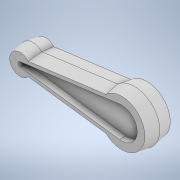
# Autodesk Inventor part: Ch3 Part 2
Saved by Autodesk Inventor 2020 (Build 240168000, 168)
## iProperties
Created: 2021-02-04
Part Number: Ch3 Part 2
Material: Generic
Document SubType Name: Modeling
Designer: austi
Density: 1 g/cm^3
Appearance: Default
Author: austi
Autodesk Inventor part; units mm, degrees
ref_plane "YZ Plane" through (0, 0, 0) normal (1, 0, 0) x (0, 1, 0)
ref_plane "XZ Plane" through (0, 0, 0) normal (0, 1, 0) x (-1, 0, 0)
ref_plane "XY Plane" through (0, 0, 0) normal (0, 0, 1) x (1, 0, 0)
sketch "Sketch1" plane through (0, 0, 0) normal (0, 0, 1) x (1, 0, 0)
  line L0 (-40.64, 0) -> (154.94, 0)
  line L1 (0, -35.56) -> (0, 35.56)
  arc A0 (8.901936, 9.057899) -> (8.901936, -9.057899) centre (0, 0) ccw
  arc A1 (84.799479, -19.05) -> (84.799479, 19.05) centre (101.6, 0) ccw
  line L2 (8.901936, 9.057899) -> (84.799479, 19.05)
  line L3 (8.901936, -9.057899) -> (84.799479, -19.05)
  dimension "d1" = 25.4
  dimension "d3" = 50.8
  dimension "d4" = 15
  dimension "d5" = 38.1
  dimension "d6" = 101.6
  constraints: 4 end point, 4 point on circle, 2 centre point, 2 vertical alignment, 1 coincident, 1 horizontal alignment
  measures "d1" diameter of A0
  measures "d3" diameter of A1
  measures "d4" angle of L3 L2
  measures "d5" distance of L3.end L2.end
  measures "d6" distance of A1.centre point (0, 0)
sketch "Sketch1 outline for Extrusion1" plane through (0, 0, 0) normal (0, 0, 1) x (1, 0, 0)
  arc A0 (8.901936, 9.057899) -> (8.901936, -9.057899) centre (0, 0) ccw
  line L0 (84.799479, 19.05) -> (8.901936, 9.057899)
  arc A1 (84.799479, -19.05) -> (84.799479, 19.05) centre (101.6, 0) ccw
  line L1 (8.901936, -9.057899) -> (84.799479, -19.05)
extrude "Extrusion1" add sketch "Sketch1 outline for Extrusion1" along normal mid plane 25.4 draft -10
sketch "Sketch2" plane through (0, 0, 12.7) normal (0, 0, 1) x (1, 0, 0)
  line L0 (0, 2.296768) -> (99.571808, 15.405645)
  line L1 (8.044726, 6.686369) -> (85.785782, 16.921173)
  line L2 (0, -35.56) -> (0, 35.56)
  line L3 (-40.64, 0) -> (154.94, 0)
  line L4 (0, -2.296768) -> (99.571808, -15.405645)
  arc A0 (0, 2.296768) -> (0, -2.296768) centre (0.302375, 0) ccw
  arc A1 (99.571808, -15.405645) -> (99.571808, 15.405645) centre (101.6, 0) ccw
  arc A2 (85.785782, -16.921173) -> (85.785782, 16.921173) centre (101.6, 0) ccw
  point P0 (0, 0)
  point P1 (8.355059, 3.396732)
  point P2 (8.355059, -3.396732)
  dimension "d10" = 3.302
  constraints: 6 point on line, 4 end point, 4 point on circle, 2 centre point, 2 symmetric about line, 2 tangent, 1 concentric, 1 parallel
  measures "d10" distance between parallel lines of L1 L0
extrude "Extrusion2" cut sketch "Sketch2" against normal blind 6.35
sketch "Sketch3" plane through (0, 0, -12.7) normal (0, 0, -1) x (-1, 0, 0)
  arc A0 (0, -2.296768) -> (0, 2.296768) centre (-0.302375, 0) ccw
  arc A1 (0, -2.296768) -> (0, 2.296768) centre (-0.302375, 0) ccw
  line L0 (-99.571808, -15.405645) -> (0, -2.296768)
  line L1 (0, 2.296768) -> (-99.571808, 15.405645)
  arc A2 (-99.571808, 15.405645) -> (-99.571808, -15.405645) centre (-101.6, 0) ccw
  arc A3 (-99.571808, 15.405645) -> (-99.571808, -15.405645) centre (-101.6, 0) ccw
  line L2 (0, -2.296768) -> (-99.571808, -15.405645)
  line L3 (-85.785782, 16.921173) -> (-8.044726, 6.686369)
  point P0 (0, 0)
  point P1 (0, 2.296768)
  constraints: 6 end point, 5 point on circle, 2 centre point, 2 coincident, 1 collinear, 1 parallel, 1 point on line
extrude "Extrusion3" cut sketch "Sketch3" against normal blind 6.35
body "Solid1"
